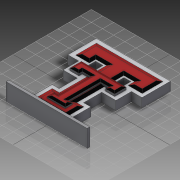
# Autodesk Inventor part: TexasTechLogo
Saved by Autodesk Inventor 2015 (Build 190159000, 159)
## iProperties
Created: 2015-05-20
Part Number: TexasTechLogo
Material: Generic
Document SubType Name: Modeling
Designer: Yeyo
Density: 1 g/cm^3
Appearance: Default
Author: Yeyo
Autodesk Inventor part; units mm, degrees
ref_plane "YZ Plane" through (0, 0, 0) normal (1, 0, 0) x (0, 1, 0)
ref_plane "XZ Plane" through (0, 0, 0) normal (0, 1, 0) x (-1, 0, 0)
ref_plane "XY Plane" through (0, 0, 0) normal (0, 0, 1) x (1, 0, 0)
sketch "Sketch1" plane through (0, 0, 0) normal (0, 1, 0) x (-1, 0, 0)
  line L0 (145.27241, -105.736161) -> (-143.65259, -105.736161) construction
  line L1 (-143.65259, -105.736161) -> (-143.65259, 111.010512) construction
  line L2 (-143.65259, 111.010512) -> (145.27241, 111.010512) construction
  line L3 (145.27241, 111.010512) -> (145.27241, -105.736161) construction
  line L4 (85.158037, -96.397789) -> (-83.615421, -96.397789)
  line L5 (-83.615421, -96.397789) -> (-83.615421, -31.617032)
  line L6 (-83.615421, -31.617032) -> (-59.629242, -31.617032)
  line L7 (-59.629242, -31.617032) -> (-59.629242, 3.695955)
  line L8 (-59.629242, 3.695955) -> (-27.314529, 3.695955)
  line L9 (-27.314529, 3.695955) -> (-27.314529, 44.884192)
  line L10 (-27.314529, 44.884192) -> (-43.471885, 44.884192)
  line L11 (-43.471885, 44.884192) -> (-43.471885, 101.552017)
  line L12 (-43.471885, 101.552017) -> (44.504163, 101.552017)
  line L13 (44.504163, 101.552017) -> (44.504163, 44.884192)
  line L14 (44.504163, 44.884192) -> (28.437423, 44.884192)
  line L15 (28.437423, 44.884192) -> (28.437423, 3.695955)
  line L16 (28.437423, 3.695955) -> (60.731957, 3.695955)
  line L17 (60.731957, 3.695955) -> (60.731957, -31.617032)
  line L18 (60.731957, -31.617032) -> (85.158037, -31.617032)
  line L19 (85.158037, -31.617032) -> (85.158037, -96.397789)
  line L20 (60.731957, -31.617032) -> (24.08876, -31.617032)
  line L21 (24.08876, -31.617032) -> (24.08876, -50.478823)
  line L22 (24.08876, -50.478823) -> (40.786033, -50.478823)
  line L23 (40.786033, -50.478823) -> (40.786033, -36.045588)
  line L24 (40.786033, -36.045588) -> (40.786033, -31.617032)
  line L25 (-59.629242, -31.617032) -> (-23.739023, -31.617032)
  line L26 (-23.739023, -31.617032) -> (-23.739023, -50.478823)
  line L27 (-23.739023, -50.478823) -> (-39.304278, -50.478823)
  line L28 (-39.304278, -50.478823) -> (-39.304278, -31.617032)
  point P0 (0, 0)
  constraints: 50 end point, 17 perpendicular, 12 point on line, 2 horizontal, 2 other
extrude "Extrusion1" add sketch "Sketch1" along normal blind 20
sketch "Sketch2" plane through (0, 20, 0) normal (0, 1, 0) x (1, 0, 0)
  line L0 (-51.542826, 2.58777) -> (-30.864745, 2.58777)
  line L1 (-30.864745, 2.58777) -> (-30.864745, 10.23619)
  line L2 (-51.542826, 29.029918) -> (-51.542826, 2.58777)
  line L3 (29.76203, 2.58777) -> (50.440111, 2.58777)
  line L4 (50.440111, 2.58777) -> (50.440111, 29.029918)
  line L5 (29.76203, 10.23619) -> (29.76203, 2.58777)
  line L6 (10.353069, 10.23619) -> (10.353069, -63.064995)
  line L7 (-11.455784, -63.064995) -> (-11.455784, 10.23619)
  line L8 (20.187472, -63.064995) -> (20.187472, -79.415179)
  line L9 (20.187472, -79.415179) -> (-21.290186, -79.415179)
  line L10 (-21.290186, -79.415179) -> (-21.290186, -63.064995)
  line L11 (29.76203, 10.23619) -> (10.353069, 10.23619)
  line L12 (-11.455784, 10.23619) -> (-30.864745, 10.23619)
  line L13 (-21.290186, -63.064995) -> (-11.455784, -63.064995)
  line L14 (10.353069, -63.064995) -> (20.187472, -63.064995)
  line L15 (50.440111, 29.029918) -> (-51.542826, 29.029918)
  line L16 (59.629242, -3.695955) -> (59.629242, 31.617032)
  line L17 (-60.731957, 31.617032) -> (-60.731957, -3.695955)
  point P0 (0, 0)
  dimension "d71" = 9.8344
  dimension "d72" = 9.8344
  dimension "d74" = 20.67808
  dimension "d75" = 20.67808
  dimension "d76" = 19.40896
  dimension "d77" = 19.40896
  dimension "d78" = 9.18913
  dimension "d79" = 9.18913
  constraints: 32 end point, 6 parallel, 5 horizontal, 4 perpendicular, 1 collinear, 1 point on line
  measures "d71" distance of L6.end L8.start
  measures "d72" distance of L10.end L7.start
  measures "d74" distance of L0.start L0.end
  measures "d75" distance of L3.start L3.end
  measures "d76" distance of L5.start L6.start
  measures "d77" distance of L7.end L1.end
  measures "d78" distance between parallel lines of L16 L4
  measures "d79" distance between parallel lines of L17 L2
sketch "Sketch3" plane through (0, 20, 0) normal (0, 1, 0) x (1, 0, 0)
  line L0 (-145.457015, 105.38773) -> (143.467985, 105.38773) construction
  line L1 (143.467985, 105.38773) -> (143.467985, -111.358944) construction
  line L2 (143.467985, -111.358944) -> (-145.457015, -111.358944) construction
  line L3 (-145.457015, -111.358944) -> (-145.457015, 105.38773) construction
  line L4 (-75.564462, 87.091249) -> (75.930391, 87.091249)
  line L5 (75.930391, 87.091249) -> (75.930391, 54.523513)
  line L6 (-75.564462, 54.523513) -> (-75.564462, 87.091249)
  line L7 (43.728587, 39.886328) -> (75.930391, 39.886328)
  line L8 (75.930391, 39.886328) -> (75.930391, 87.091249)
  line L9 (75.930391, 87.091249) -> (43.728587, 87.091249)
  line L10 (43.728587, 54.523513) -> (43.728587, 39.886328)
  line L11 (-75.564462, 39.886328) -> (-44.460446, 39.886328)
  line L12 (-44.460446, 39.886328) -> (-44.460446, 54.523513)
  line L13 (-44.460446, 87.091249) -> (-75.564462, 87.091249)
  line L14 (-75.564462, 87.091249) -> (-75.564462, 39.886328)
  line L15 (19.211304, 54.523513) -> (19.211304, -52.693865)
  line L16 (-19.943163, -52.693865) -> (-19.943163, 54.523513)
  line L17 (35.678136, -52.693865) -> (35.678136, -94.043912)
  line L18 (35.678136, -94.043912) -> (-36.409995, -94.043912)
  line L19 (-36.409995, -94.043912) -> (-36.409995, -52.693865)
  line L20 (43.728587, 54.523513) -> (19.211304, 54.523513)
  line L21 (-19.943163, 54.523513) -> (-44.460446, 54.523513)
  line L22 (-36.409995, -52.693865) -> (-19.943163, -52.693865)
  line L23 (19.211304, -52.693865) -> (35.678136, -52.693865)
  point P0 (0, 0)
  constraints: 40 end point, 11 parallel, 5 horizontal, 5 perpendicular, 3 point on line, 2 other
extrude "Extrusion2" add sketch "Sketch3" along normal blind 2 draft -75
extrude "Extrusion3" add sketch "Sketch2" along normal blind 5
sketch "Sketch4" plane through (0, 25, 0) normal (0, 1, 0) x (1, 0, 0)
  line L0 (-51.55313, 2.58777) -> (-30.864745, 2.58777)
  line L1 (-30.864745, 2.58777) -> (-30.864745, 10.23619)
  line L2 (-51.55313, 29.029918) -> (-51.55313, 2.58777)
  line L3 (29.76203, 2.58777) -> (50.440111, 2.58777)
  line L4 (50.440111, 2.58777) -> (50.440111, 29.029918)
  line L5 (29.76203, 10.23619) -> (29.76203, 2.58777)
  line L6 (10.353069, 10.23619) -> (10.353069, -63.064995)
  line L7 (-11.455784, -63.064995) -> (-11.455784, 10.23619)
  line L8 (20.187472, -63.064995) -> (20.187472, -79.415179)
  line L9 (20.187472, -79.415179) -> (-21.290186, -79.415179)
  line L10 (-21.290186, -79.415179) -> (-21.290186, -63.064995)
  line L11 (29.76203, 10.23619) -> (10.353069, 10.23619)
  line L12 (-11.455784, 10.23619) -> (-30.864745, 10.23619)
  line L13 (-21.290186, -63.064995) -> (-11.455784, -63.064995)
  line L14 (10.353069, -63.064995) -> (20.187472, -63.064995)
  line L15 (50.440111, 29.029918) -> (-51.55313, 29.029918)
  line L16 (-30.864745, 10.23619) -> (-11.455784, 10.23619)
  line L17 (-11.455784, 10.23619) -> (-11.455784, -63.064995)
  line L18 (10.353069, -63.064995) -> (10.353069, 10.23619)
  line L19 (-21.290186, -63.064995) -> (-21.290186, -79.415179)
  line L20 (-51.542826, 2.58777) -> (-30.864745, 2.58777)
  line L21 (50.440111, 2.58777) -> (50.440111, 29.029918)
  line L22 (29.76203, 10.23619) -> (29.76203, 2.58777)
  line L23 (-30.864745, 2.58777) -> (-30.864745, 10.23619)
  line L24 (20.187472, -79.415179) -> (20.187472, -63.064995)
  point P0 (0, 0)
  point P1 (0, 0)
  constraints: 32 end point, 10 collinear, 6 parallel, 5 horizontal, 4 perpendicular, 1 point on line
sketch "Sketch4 outline for Extrusion4" plane through (0, 25, 0) normal (0, 1, 0) x (1, 0, 0)
  line L0 (-51.55313, 29.029918) -> (-51.55313, 2.58777)
  line L1 (50.440111, 29.029918) -> (-51.55313, 29.029918)
  line L2 (50.440111, 2.58777) -> (50.440111, 29.029918)
  line L3 (29.76203, 2.58777) -> (50.440111, 2.58777)
  line L4 (29.76203, 10.23619) -> (29.76203, 2.58777)
  line L5 (10.353069, 10.23619) -> (29.76203, 10.23619)
  line L6 (10.353069, -63.064995) -> (10.353069, 10.23619)
  line L7 (20.187472, -63.064995) -> (10.353069, -63.064995)
  line L8 (20.187472, -79.415179) -> (20.187472, -63.064995)
  line L9 (-21.290186, -79.415179) -> (20.187472, -79.415179)
  line L10 (-21.290186, -63.064995) -> (-21.290186, -79.415179)
  line L11 (-11.455784, -63.064995) -> (-21.290186, -63.064995)
  line L12 (-11.455784, 10.23619) -> (-11.455784, -63.064995)
  line L13 (-30.864745, 10.23619) -> (-11.455784, 10.23619)
  line L14 (-30.864745, 2.58777) -> (-30.864745, 10.23619)
  line L15 (-51.55313, 2.58777) -> (-30.864745, 2.58777)
extrude "Extrusion4" add sketch "Sketch4 outline for Extrusion4" along normal blind 2 draft -70
sketch "Sketch5" plane through (0, 20, 0) normal (0, 1, 0) x (1, 0, 0)
  line L0 (-92.761717, -95.552017) -> (91.729439, -95.552017)
  line L1 (91.729439, -95.552017) -> (91.729439, -101.552017)
  line L2 (91.729439, -101.552017) -> (-92.761717, -101.552017)
  line L3 (-92.761717, -101.552017) -> (-92.761717, -95.552017)
  line L4 (-44.504163, -101.552017) -> (43.471885, -101.552017)
  line L5 (-44.504163, -44.884192) -> (-44.504163, -101.552017)
  line L6 (43.471885, -101.552017) -> (43.471885, -44.884192)
  point P0 (0, 0)
  dimension "d58" = 48.25755
  dimension "d59" = 48.25755
  dimension "d60" = 6
  constraints: 8 end point, 2 parallel, 1 collinear, 1 horizontal, 1 perpendicular
  measures "d58" distance between parallel lines of L5 L3
  measures "d59" distance between parallel lines of L1 L6
  measures "d60" distance between parallel lines of L2 L0
extrude "Extrusion5" add sketch "Sketch5" along normal blind 10 and the other way blind 30
equation "\"d72\" = d71"
equation "\"d75\" = d74"
equation "\"d77\" = d76"
equation "\"d79\" = d78"
equation "\"d59\" = d58"
body "Solid1"
